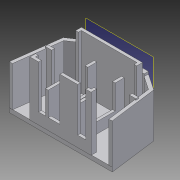
# Autodesk Inventor part: conrad_schaltsteckdose
Saved by Autodesk Inventor 2012 (Build 160160000, 160)
## iProperties
Created: 2013-07-23
Part Number: conrad_schaltsteckdose
Material: Default
Document SubType Name: Modeling
Designer: befi
Density: 1 g/cm^3
Author: befi
Autodesk Inventor part; units mm, degrees
ref_plane "YZ Plane" through (0, 0, 0) normal (1, 0, 0) x (0, 1, 0)
ref_plane "XZ Plane" through (0, 0, 0) normal (0, 1, 0) x (-1, 0, 0)
ref_plane "XY Plane" through (0, 0, 0) normal (0, 0, 1) x (1, 0, 0)
sketch "Skizze1" plane through (0, 0, 0) normal (0, 0, 1) x (1, 0, 0)
  line L0 (-20.9977, -1.3) -> (5.0023, -1.3)
  line L1 (-22.2477, 0) -> (6.2523, 0)
  line L2 (-22.2477, 0) -> (-22.2477, -2.7)
  line L3 (-22.2477, -2.7) -> (-20.9977, -2.7)
  line L4 (-20.9977, -2.7) -> (-20.9977, -1.3)
  line L5 (5.0023, -1.3) -> (5.0023, -2.7)
  line L6 (5.0023, -2.7) -> (6.2523, -2.7)
  line L7 (6.2523, -2.7) -> (6.2523, 0)
  point P0 (0, 0)
  dimension "d0" = 26
  dimension "d1" = 28.5
  dimension "d2" = 1.25
  dimension "d33" = 1.3
  dimension "d37" = 2.7
  dimension "d38" = 2.7
  dimension "d39" = 0
  constraints: 16 end point, 4 parallel, 3 perpendicular, 1 horizontal
  measures "d0" distance of L0.start L0.end
  measures "d1" distance of L1.start L1.end
  measures "d2" distance of L2.end L3.end
  measures "d33" distance between parallel lines of L1 L0
  measures "d37" distance of L6.end L1.end
  measures "d38" distance of L1.start L2.end
  measures "d39" distance from line of L1 point (0, 0)
extrude "Extrusion1" add sketch "Skizze1" along normal blind 25.5
sketch "Skizze2" plane through (0, 0, 0) normal (0, 0, -1) x (-1, 0, 0)
  line L0 (20.9977, -1.3) -> (-5.0023, -1.3) projected
  line L1 (20.9977, -2.7) -> (20.9977, -1.3) projected
  line L2 (-5.0023, -1.3) -> (-5.0023, -2.7) projected
  line L3 (0.9977, -1.3) -> (2.2477, -1.3)
  line L4 (2.2477, -1.3) -> (2.2477, -5.5195)
  line L5 (2.2477, -5.5195) -> (0.9977, -5.5195)
  line L6 (0.9977, -5.5195) -> (0.9977, -1.3)
  line L7 (13.7477, -1.3) -> (14.9977, -1.3)
  line L8 (14.9977, -1.3) -> (14.9977, -5.5195)
  line L9 (14.9977, -5.5195) -> (13.7477, -5.5195)
  line L10 (13.7477, -5.5195) -> (13.7477, -1.3)
  point P0 (0, 0)
  dimension "d5" = 11.5
  dimension "d6" = 1.25
  dimension "d7" = 1.25
  dimension "d8" = 6
  dimension "d9" = 6
  constraints: 16 end point, 4 parallel, 2 horizontal, 2 perpendicular, 2 point on line
  measures "d5" distance between parallel lines of L10 L4
  measures "d6" distance of L4.end L5.end
  measures "d7" distance of L8.end L9.end
  measures "d8" distance between parallel lines of L2 L6
  measures "d9" distance between parallel lines of L1 L8
extrude "Extrusion2" add sketch "Skizze2" against normal blind 16.35
sketch "Skizze3" plane through (0, 0, 0) normal (0, 0, -1) x (-1, 0, 0)
  line L0 (0.9977, -5.5195) -> (2.2477, -5.5195)
  line L1 (2.2477, -5.5195) -> (2.2477, -17.7695)
  line L2 (2.2477, -17.7695) -> (0.9977, -17.7695)
  line L3 (0.9977, -17.7695) -> (0.9977, -5.5195)
  line L4 (13.7477, -5.5195) -> (14.9977, -5.5195)
  line L5 (14.9977, -5.5195) -> (14.9977, -17.7695)
  line L6 (14.9977, -17.7695) -> (13.7477, -17.7695)
  line L7 (13.7477, -17.7695) -> (13.7477, -5.5195)
  point P0 (0, 0)
  dimension "d12" = 12.25
  dimension "d15" = 12.25
  constraints: 16 end point, 4 parallel, 2 horizontal, 2 perpendicular
  measures "d12" distance of L2.end L0.start
  measures "d15" distance of L4.end L5.end
extrude "Extrusion3" add sketch "Skizze3" against normal blind 5
sketch "Skizze4" plane through (0, 0, 0) normal (0, 0, -1) x (-1, 0, 0)
  line L0 (0.9977, -17.7695) -> (2.2477, -17.7695)
  line L1 (2.2477, -17.7695) -> (2.2477, -24.0195)
  line L2 (2.2477, -24.0195) -> (0.9977, -24.0195)
  line L3 (0.9977, -24.0195) -> (0.9977, -17.7695)
  line L4 (13.7477, -17.7695) -> (14.9977, -17.7695)
  line L5 (14.9977, -17.7695) -> (14.9977, -24.0195)
  line L6 (14.9977, -24.0195) -> (13.7477, -24.0195)
  line L7 (13.7477, -24.0195) -> (13.7477, -17.7695)
  point P0 (0, 0)
  dimension "d16" = 6.25
  dimension "d17" = 6.25
  constraints: 16 end point, 4 parallel, 2 horizontal, 2 perpendicular
  measures "d16" distance of L2.end L0.start
  measures "d17" distance of L6.end L4.start
extrude "Extrusion4" add sketch "Skizze4" against normal blind 16.35
sketch "Skizze5" plane through (-14.9977, -24.0195, 0) normal (0, -1, 0) x (1, 0, 0)
  line L0 (-7.25, 0) -> (-7.25, 25.5) projected
  line L1 (21.25, 0) -> (21.25, 25.5) projected
  line L2 (-7.25, 25.5) -> (-7.25, 0)
  line L3 (21.25, 0) -> (-7.25, 0)
  line L4 (21.25, 0) -> (21.25, 25.5)
  line L5 (21.25, 25.5) -> (18.8, 25.5)
  line L6 (18.8, 25.5) -> (18.8, 5.0223)
  line L7 (18.8, 5.0223) -> (15, 5.0223)
  line L8 (15, 5.0223) -> (15, 25.5)
  line L9 (15, 25.5) -> (6.75, 25.5)
  line L10 (6.75, 25.5) -> (6.75, 5.25)
  line L11 (6.75, 5.25) -> (-3.25, 5.25)
  line L12 (-3.25, 5.25) -> (-3.25, 25.5)
  line L13 (-3.25, 25.5) -> (-7.25, 25.5)
  point P0 (14.9977, 0)
  dimension "d20" = 5.25
  dimension "d21" = 8.25
  dimension "d22" = 3.8
  dimension "d23" = 10
  dimension "d24" = 4
  dimension "d25" = 2.45
  constraints: 24 end point, 6 parallel, 4 collinear, 3 perpendicular
  measures "d20" distance between parallel lines of L3 L11
  measures "d21" distance of L8.end L9.end
  measures "d22" distance of L6.end L7.end
  measures "d23" distance of L10.end L11.end
  measures "d24" distance of L12.end L0.end
  measures "d25" distance of L1.end L5.end
extrude "Extrusion5" add sketch "Skizze5" against normal blind 1.3
sketch "Skizze6" plane through (-14.9977, -22.7195, 0) normal (0, 1, 0) x (1, 0, 0)
  line L0 (-3.25, -25.5) -> (-7.25, -25.5) projected
  line L1 (14, 0) -> (21.25, 0) projected
  line L2 (21.25, -25.5) -> (21.25, 0)
  line L3 (-7.25, 0) -> (-6, 0)
  line L4 (-6, 0) -> (-6, -25.5)
  line L5 (-6, -25.5) -> (-7.25, -25.5)
  line L6 (-7.25, -25.5) -> (-7.25, 0)
  line L7 (21.25, 0) -> (20, 0)
  line L8 (20, 0) -> (20, -25.5)
  line L9 (20, -25.5) -> (21.25, -25.5)
  line L10 (21.25, -25.5) -> (21.25, 0)
  point P0 (14.9977, 0)
  point P1 (18.8, -25.5)
  dimension "d28" = 1.25
  dimension "d30" = 1.25
  constraints: 18 end point, 4 parallel, 2 horizontal, 2 perpendicular, 1 point on line
  measures "d28" distance of L4.end L5.end
  measures "d30" distance of L9.end L8.end
extrude "Extrusion6" add sketch "Skizze6" along normal blind 1.3
sketch "Skizze7" plane through (0, 0, 0) normal (0, 0, -1) x (-1, 0, 0)
  line L0 (22.2477, 0) -> (22.2477, -2.7) projected
  line L1 (-6.2523, -2.7) -> (-6.2523, 0) projected
  line L2 (-13.1523, -8.7) -> (-10.1523, -8.7)
  line L3 (-10.1523, -8.7) -> (-10.1523, -10)
  line L4 (-10.1523, -10) -> (-13.1523, -10)
  line L5 (-13.1523, -10) -> (-13.1523, -8.7)
  line L6 (26.1477, -8.7) -> (29.1477, -8.7)
  line L7 (29.1477, -8.7) -> (29.1477, -10)
  line L8 (29.1477, -10) -> (26.1477, -10)
  line L9 (26.1477, -10) -> (26.1477, -8.7)
  line L10 (22.2477, -2.7) -> (20.9977, -2.7) projected
  line L11 (-5.0023, -2.7) -> (-6.2523, -2.7) projected
  point P0 (0, 0)
  dimension "d40" = 3.9
  dimension "d41" = 3.9
  dimension "d42" = 1.3
  dimension "d43" = 3
  dimension "d44" = 3
  dimension "d45" = 1.3
  dimension "d68" = 6
  dimension "d69" = 6
  constraints: 16 end point, 4 parallel, 2 horizontal, 2 perpendicular
  measures "d40" distance from line of L3.end L1
  measures "d41" distance between parallel lines of L0 L9
  measures "d42" distance of L4.end L2.start
  measures "d43" distance of L3.end L4.end
  measures "d44" distance of L7.end L8.end
  measures "d45" distance of L6.end L7.end
  measures "d68" distance between parallel lines of L11 L2
  measures "d69" distance between parallel lines of L10 L6
extrude "Extrusion7" add sketch "Skizze7" against normal blind 19.3
ref_plane "Arbeitsebene1" through (-22.2477, 3.5, 0) normal (0, 1, 0) x (1, 0, 0)
sketch "Skizze9" plane through (-22.2477, 3.5, 0) normal (0, 1, 0) x (1, 0, 0)
  line L0 (28.5, 0) -> (28.5, -25.5)
  line L1 (28.5, 0) -> (0, 0)
  line L2 (0, 0) -> (0, -25.5)
  line L3 (0.75, 0) -> (27.75, 0)
  line L4 (27.75, 0) -> (27.75, -19.8)
  line L5 (27.75, -19.8) -> (0.75, -19.8)
  line L6 (0.75, -19.8) -> (0.75, 0)
  point P0 (22.2477, 0)
  point P1 (22.2477, 0)
  dimension "d55" = 27
  dimension "d56" = 19.8
  dimension "d57" = 0.75
  dimension "d58" = 0.75
  constraints: 14 end point, 2 parallel, 1 horizontal, 1 perpendicular, 1 point on line
  measures "d55" distance of L4.end L5.end
  measures "d56" distance of L5.end L3.start
  measures "d57" distance between parallel lines of L2 L6
  measures "d58" distance between parallel lines of L4 L0
extrude "Extrusion9" add sketch "Skizze9" against normal blind 2
sketch "Skizze11" plane through (0, 0, 0) normal (0, 0, -1) x (-1, 0, 0)
  line L0 (22.2477, -24.0195) -> (22.2477, -21.4195) projected
  line L1 (22.2477, 0) -> (22.2477, -2.7) projected
  line L2 (-6.2523, -2.7) -> (-6.2523, 0) projected
  line L3 (-6.2523, -24.0195) -> (-6.2523, -21.4195) projected
  line L4 (-11.7523, -2.7) -> (-14.5023, -24.0195)
  line L5 (27.7477, -2.7) -> (30.4977, -24.0195)
  line L6 (-5.5023, 3.5) -> (-5.5023, 1.5) projected
  line L7 (21.4977, 3.5) -> (21.4977, 1.5) projected
  line L8 (-11.7523, -2.7) -> (-5.5023, 1.5)
  line L9 (-5.5023, 1.5) -> (-5.5023, 3.5)
  line L10 (27.7477, -2.7) -> (21.4977, 1.5)
  line L11 (21.4977, 1.5) -> (21.4977, 3.5)
  line L12 (21.4977, 3.5) -> (29.1227, -1.624)
  line L13 (29.1227, -1.624) -> (31.9868, -23.8275)
  line L14 (31.9868, -23.8275) -> (30.4977, -24.0195)
  line L15 (-5.5023, 1.5) -> (-5.5023, 3.5)
  line L16 (-5.5023, 3.5) -> (-13.1273, -1.624)
  line L17 (-13.1273, -1.624) -> (-15.9913, -23.8275)
  line L18 (-15.9913, -23.8275) -> (-14.5023, -24.0195)
  point P0 (0, 0)
  dimension "d65" = 28.5
  dimension "d66" = 8.25
  dimension "d67" = 8.25
  dimension "d70" = 5.5
  dimension "d71" = 5.5
  constraints: 26 end point, 5 parallel, 2 perpendicular, 1 collinear
  measures "d65" distance of L3.start L0.start
  measures "d66" distance from line of L3 L4.end
  measures "d67" distance from line of L5.end L0
  measures "d70" distance from line of L2 L4.start
  measures "d71" distance from line of L1 L5.start
extrude "Extrusion10" add sketch "Skizze11" against normal blind 18.7
sketch "Skizze12" plane through (0, 0, 0) normal (0, 0, -1) x (-1, 0, 0)
  line L0 (31.9868, -23.8275) -> (29.1227, -1.624) projected
  line L1 (29.1227, -1.624) -> (21.4977, 3.5) projected
  line L2 (21.4977, 3.5) -> (-5.5023, 3.5) projected
  line L3 (-5.5023, 3.5) -> (-13.1273, -1.624) projected
  line L4 (-13.1273, -1.624) -> (-15.9913, -23.8275) projected
  line L5 (-15.9913, -23.8275) -> (31.9868, -23.8275)
  point P0 (0, 0)
  constraints: 2 end point
extrude "Extrusion11" add sketch "Skizze12" along normal blind 2
equation "\"d38\" = d37"
equation "\"d7\" = d6"
equation "\"d15\" = d12"
equation "\"d17\" = d16"
equation "\"d41\" = d40"
equation "\"d44\" = d43"
equation "\"d45\" = d42"
equation "\"d69\" = d68"
equation "\"d57\" = d58"
equation "\"d66\" = d67"
equation "\"d70\" = d71"
